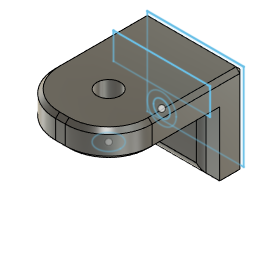
Arm Mount (Autodesk Fusion 360 design; units mm, degrees)
Autodesk Fusion 360 part; units mm, degrees
sketch "sketch 680" plane through (0, 380, 0) normal (0, -1, 0) x (1, 0, 0)
  line L0 (-185.0624, -39) -> (-185.0624, -21)
  line L1 (-185.0624, -21) -> (-205.0624, -21)
  line L2 (-185.0624, -21) -> (-205.0624, -21)
  line L3 (-205.0624, -21) -> (-205.0624, -39)
  line L4 (-205.0624, -39) -> (-185.0624, -39)
extrude "Extrude1" add sketch "sketch 680" along normal blind 7
sketch "sketch 730" plane through (0, 373, 0) normal (0, -1, 0) x (1, 0, 0)
  line L0 (-185.0624, -26.5) -> (-205.0624, -26.5)
  line L1 (-185.0624, -21) -> (-185.0624, -26.5)
  line L2 (-185.0624, -21) -> (-185.0624, -26.5)
  line L3 (-205.0624, -21) -> (-185.0624, -21)
  line L4 (-205.0624, -21) -> (-185.0624, -21)
  line L5 (-205.0624, -26.5) -> (-205.0624, -21)
  line L6 (-205.0624, -26.5) -> (-205.0624, -21)
extrude "Extrude4" add sketch "sketch 730" along normal blind 21
sketch "sketch 715" plane through (0, 373, 0) normal (0, -1, 0) x (1, 0, 0)
  circle A0 centre (-195.0624, -30) radius 1.7
  circle A1 centre (-195.0624, -30) radius 3
extrude "Extrude3" cut sketch "sketch 715" against normal blind 3
sketch "sketch 703" plane through (0, 373, 0) normal (0, -1, 0) x (1, 0, 0)
  circle A0 centre (-195.0624, -30) radius 1.7
extrude "Extrude2" cut sketch "sketch 703" against normal blind 7
sketch "sketch 754" plane through (0, 0, -30.5) normal (0, 0, -1) x (1, 0, 0)
  circle A0 centre (-195.0624, -362) radius 2.425
extrude "Extrude5" cut sketch "sketch 754" against normal blind 10
fillet "Fillet1" radius 9 2 edges at (-185.0624, 352, -23.75) (-205.0624, 352, -23.75)
chamfer "Chamfer1" distance 0.8 angle 45 10 edges at (-205.0624, 370.5, -21) (-202.4264, 354.636, -21) (-195.0624, 352, -21) (-187.6985, 354.636, -21) (-185.0624, 370.5, -21) (-205.0624, 367, -26.5) (-202.4264, 354.636, -26.5) (-195.0624, 352, -26.5) (-187.6985, 354.636, -26.5) (-185.0624, 367, -26.5) 1 faces at (-202.2958, 380, -30)
chamfer "Chamfer2" distance 2 angle 45 3 edges at (-205.0624, 373, -32.75) (-195.0624, 373, -39) (-185.0624, 373, -32.75)
fillet "Fillet2" radius 2 3 edges at (-203.0624, 373, -31.75) (-195.0624, 373, -37) (-187.0624, 373, -31.75)
named bodies: "Tube mount"
